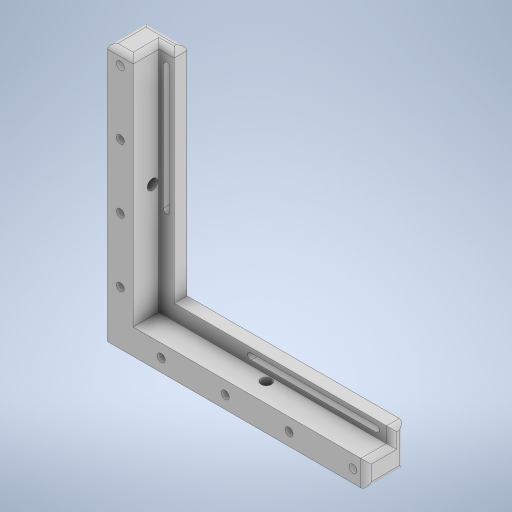
# Autodesk Inventor part: DUT Holder v1.0
Saved by Autodesk Inventor 2024 (Build 280153000, 153)
## iProperties
Created: 2024-09-24
Part Number: DUT Holder v1.0
Material: Generic
Document SubType Name: Modeling
Designer: Kemper Room 121
Density: 1 g/cm^3
Appearance: Default
Author: Kemper Room 121
Autodesk Inventor part; units mm, degrees
ref_plane "YZ Plane" through (0, 0, 0) normal (1, 0, 0) x (0, 1, 0)
ref_plane "XZ Plane" through (0, 0, 0) normal (0, 1, 0) x (-1, 0, 0)
ref_plane "XY Plane" through (0, 0, 0) normal (0, 0, 1) x (1, 0, 0)
sketch "Sketch1" plane through (0, 0, 0) normal (0, 0, 1) x (1, 0, 0)
  line L0 (0, 0) -> (0, 101)
  line L1 (0, 101) -> (10, 101)
  line L2 (10, 101) -> (16, 101)
  line L3 (16, 101) -> (16, 16)
  line L4 (16, 16) -> (101, 16)
  line L5 (101, 16) -> (101, 0)
  line L6 (101, 0) -> (0, 0)
  line L7 (16, 101) -> (13, 101)
  line L8 (13, 101) -> (13, 13)
  line L9 (13, 13) -> (101, 13)
  line L10 (16, 16) -> (13, 16)
  line L11 (16, 16) -> (16, 13)
  line L12 (10, 101) -> (10, 8)
  line L13 (10, 8) -> (101, 8)
  line L14 (16, 13) -> (46, 13)
  line L15 (101, 13) -> (95, 13)
  line L16 (13, 101) -> (13, 95)
  circle A0 centre (95, 13) radius 1.25
  circle A1 centre (46, 13) radius 1.25
  circle A2 centre (13, 95) radius 1.25
  line L17 (13, 16) -> (13, 46)
  circle A3 centre (13, 46) radius 1.25
  line L18 (11.75, 95) -> (11.75, 46)
  line L19 (14.25, 46) -> (14.25, 95)
  line L20 (46, 14.25) -> (95, 14.25)
  line L21 (46, 11.75) -> (95, 11.75)
  point P0 (58.5, 16)
  dimension "d0" = 101
  dimension "d1" = 10
  dimension "d2" = 6
  dimension "d3" = 101
  dimension "d4" = 16
  dimension "d32" = 3
  dimension "d34" = 3
  dimension "d35" = 30
  dimension "d36" = 6
  dimension "d37" = 6
  dimension "d38" = 2.5
  dimension "d39" = 2.5
  dimension "d40" = 2.5
  dimension "d41" = 30
  dimension "d42" = 2.5
  constraints: 44 end point, 8 point on circle, 8 point on line, 6 perpendicular, 6 tangent, 4 centre point, 4 coincident, 3 midpoint, 3 vertical, 1 horizontal, 1 parallel
  measures "d0" distance of L0.start L0.end
  measures "d1" distance of L0.end L1.end
  measures "d2" distance of L1.end L2.end
  measures "d3" distance of L5.end L0.start
  measures "d4" distance of L4.end L5.end
  measures "d32" distance of L2.end L7.end
  measures "d34" distance from line of point (58.5, 16) L9
  measures "d35" distance of L11.end L14.end
  measures "d36" distance of L9.end L15.end
  measures "d37" distance of L7.end L16.end
  measures "d38" diameter of A0
  measures "d39" diameter of A1
  measures "d40" diameter of A2
  measures "d41" distance of L10.end L17.end
  measures "d42" diameter of A3
extrude "Extrusion1" add sketch "Sketch1" along normal blind 5 contours L0 L1 L12 L13 L5 L6 | L2 L8 A2 L18 A3 L9 A1 L21 A0 L5 L13 L12 | L2 L3 L10 L8 A3 L19 A2 | L9 A0 L20 A1 L11 L4 L5 | L11 L9 L8 L10
sketch "Sketch2" plane through (0, 0, 5) normal (0, 0, 1) x (1, 0, 0)
  line L0 (101, 0) -> (101, 16) projected
  line L1 (101, 16) -> (16, 16) projected
  line L2 (16, 16) -> (16, 101) projected
  line L3 (16, 101) -> (0, 101) projected
  line L4 (0, 101) -> (0, 0) projected
  line L5 (0, 0) -> (101, 0) projected
  line L6 (0, 101) -> (10, 101)
  line L7 (10, 101) -> (10, 10)
  line L8 (10, 10) -> (101, 10)
  line L9 (101, 0) -> (101, 16) projected
  line L10 (101, 10) -> (101, 0)
  line L11 (101, 0) -> (0, 0)
  line L12 (0, 101) -> (0, 0)
  dimension "d7" = 10
  dimension "d8" = 10
  constraints: 12 end point, 3 perpendicular, 2 collinear, 2 point on line
  measures "d7" distance of L3.end L6.end
  measures "d8" distance of L0.start L8.end
extrude "Extrusion2" add sketch "Sketch2" along normal blind 10 contours L5 L4 L3 L7 L8 L0
sketch "Sketch3" plane through (0, 0, 15) normal (0, 0, 1) x (1, 0, 0)
  line L0 (10, 10) -> (10, 101) projected
  line L1 (10, 101) -> (0, 101) projected
  line L2 (0, 101) -> (0, 0) projected
  line L3 (0, 0) -> (101, 0) projected
  line L4 (101, 0) -> (101, 10) projected
  line L5 (101, 10) -> (10, 10) projected
  line L6 (0, 101) -> (5, 101)
  line L7 (5, 101) -> (5, 5)
  line L8 (5, 5) -> (101, 5)
  line L9 (10, 101) -> (10, 10) projected
  line L10 (10, 10) -> (101, 10) projected
  line L11 (101, 10) -> (101, 16) projected
  line L12 (101, 16) -> (16, 16) projected
  line L13 (16, 16) -> (16, 101) projected
  line L14 (16, 101) -> (10, 101) projected
  line L15 (5, 101) -> (5, 96)
  line L16 (5, 16) -> (5, 21)
  line L17 (16, 5) -> (21, 5)
  line L18 (101, 5) -> (96, 5)
  line L19 (5, 96) -> (5, 71)
  line L20 (5, 71) -> (5, 46)
  line L21 (21, 5) -> (46, 5)
  line L22 (46, 5) -> (71, 5)
  circle A0 centre (5, 96) radius 1.5
  circle A1 centre (5, 71) radius 1.5
  circle A2 centre (5, 46) radius 1.5
  circle A3 centre (5, 21) radius 1.5
  circle A4 centre (21, 5) radius 1.5
  circle A5 centre (46, 5) radius 1.5
  circle A6 centre (71, 5) radius 1.5
  circle A7 centre (96, 5) radius 1.5
  dimension "d11" = 5
  dimension "d12" = 5
  dimension "d13" = 85
  dimension "d14" = 5
  dimension "d15" = 5
  dimension "d16" = 5
  dimension "d17" = 5
  dimension "d18" = 25
  dimension "d19" = 25
  dimension "d20" = 25
  dimension "d21" = 25
  dimension "d22" = 3
  dimension "d23" = 3
  dimension "d24" = 3
  dimension "d25" = 3
  dimension "d26" = 3
  dimension "d27" = 3
  dimension "d28" = 3
  dimension "d29" = 3
  dimension "d47" = 25
  dimension "d48" = 25
  constraints: 22 end point, 10 point on line, 8 centre point, 8 coincident, 2 midpoint, 1 parallel
  measures "d11" distance of L1.end L6.end
  measures "d12" distance between parallel lines of L3 L8
  measures "d13" distance of L13.end L12.end
  measures "d14" distance of L6.end L15.end
  measures "d15" distance of L16.start L16.end
  measures "d16" distance of L17.start L17.end
  measures "d17" distance of L8.end L18.end
  measures "d18" distance of L15.end L19.end
  measures "d19" distance of L19.end L20.end
  measures "d20" distance of L17.end L21.end
  measures "d21" distance of L21.end L22.end
  measures "d22" diameter of A0
  measures "d23" diameter of A1
  measures "d24" diameter of A2
  measures "d25" diameter of A3
  measures "d26" diameter of A4
  measures "d27" diameter of A5
  measures "d28" diameter of A6
  measures "d29" diameter of A7
  measures "d47" distance of A2.centre A3.centre
  measures "d48" distance of L18.end L22.end
extrude "Extrusion3" cut sketch "Sketch3" against normal blind 16 contours A0 L7 | L7 A0 | A7 L8 | L8 A7 | A1 L7 | L7 A1 | A6 L8 | L8 A6 | A2 L7 | L7 A2 | A5 L8 | L8 A5 | A3 L7 | L7 A3 | A4 L8 | L8 A4
fillet "Fillet1" radius 2 11 edges at (5, 101, 15) (10, 101, 10) (16, 101, 2.5) (8, 101, 0) (0, 101, 7.5) (101, 16, 2.5) (101, 8, 0) (101, 13, 5) (101, 10, 10) (101, 5, 15) (101, 0, 7.5)
sketch "Sketch5" plane through (10, 10, 15) normal (1, 0, 0) x (0, 0, -1)
  line L0 (0, 89) -> (10, 89) projected
  line L1 (0, 0) -> (0, 89) projected
  line L2 (10, 0) -> (0, 0) projected
  line L3 (10, 89) -> (10, 0) projected
  circle A0 centre (26.9628, 94.4324) radius 2
  line L4 (0, 89) -> (10, 89) projected
  line L5 (10, 89) -> (7.5, 89)
  line L6 (7.5, 89) -> (7.5, 44.5)
  circle A1 centre (7.5, 44.5) radius 2
  point P0 (15, -10)
  dimension "d49" = 10
  dimension "d50" = 89
  dimension "d51" = 4
  dimension "d52" = 2.5
  dimension "d53" = 44.5
  dimension "d54" = 4
  constraints: 4 end point, 2 centre point, 1 coincident, 1 perpendicular, 1 point on line
  measures "d49" distance of L0.start L0.end
  measures "d50" distance of L1.start L0.start
  measures "d51" diameter of A0
  measures "d52" distance of L0.end L5.end
  measures "d53" distance of L5.end L6.end
  measures "d54" diameter of A1
extrude "Extrusion4" cut sketch "Sketch5" against normal blind 10 contours A1
sketch "Sketch6" plane through (10, 10, 15) normal (0, 1, 0) x (1, 0, 0)
  line L0 (89, 10) -> (89, 0) projected
  line L1 (0, 10) -> (89, 10) projected
  line L2 (0, 10) -> (0, 0) projected
  line L3 (89, 0) -> (0, 0) projected
  line L4 (0, 10) -> (0, 7.5)
  line L5 (0, 7.5) -> (44.5, 7.5)
  circle A0 centre (44.5, 7.5) radius 2
  point P0 (-10, 15)
  dimension "d57" = 2.5
  dimension "d58" = 44.5
  dimension "d59" = 4
  constraints: 4 end point, 1 centre point, 1 coincident, 1 perpendicular, 1 point on line
  measures "d57" distance of L1.start L4.end
  measures "d58" distance of L4.end L5.end
  measures "d59" diameter of A0
extrude "Extrusion5" cut sketch "Sketch6" against normal blind 10 contours A0
equation "\"d3\" = d0"
equation "\"d4\" = d1 + d2"
equation "\"d32\" = 0.5 * d2"
equation "\"d34\" = d32"
equation "\"d36\" = 2 * d32"
equation "\"d37\" = d36"
equation "\"d39\" = d38"
equation "\"d40\" = d38"
equation "\"d41\" = d35"
equation "\"d42\" = d38"
equation "\"d7\" = d1"
equation "\"d8\" = d1"
equation "\"d11\" = 0.5 * d1"
equation "\"d14\" = d11"
equation "\"d15\" = d11"
equation "\"d16\" = d11"
equation "\"d17\" = d11"
equation "\"d18\" = -0.666667 * d14 + 0.333333 * d13"
equation "\"d19\" = d18"
equation "\"d20\" = d18"
equation "\"d21\" = d18"
equation "\"d23\" = d22"
equation "\"d24\" = d22"
equation "\"d25\" = d22"
equation "\"d26\" = d22"
equation "\"d27\" = d22"
equation "\"d28\" = d22"
equation "\"d29\" = d22"
equation "\"d47\" = d18"
equation "\"d48\" = d18"
equation "\"d30\" = d1 + d2"
equation "\"d53\" = 0.5 * d50"
equation "\"d54\" = d51"
equation "\"d57\" = d52"
equation "\"d58\" = d53"
equation "\"d59\" = d54"
body "Solid1"
